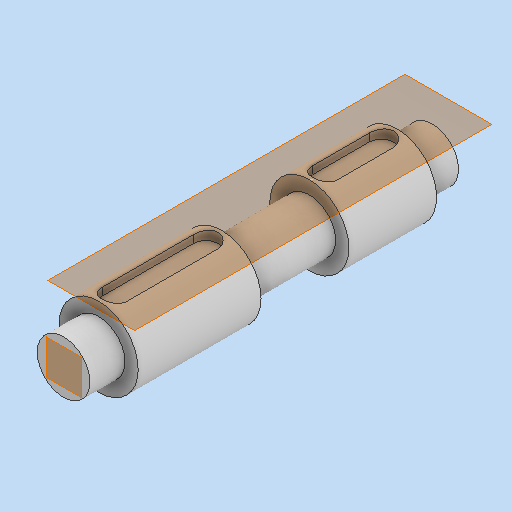
# Autodesk Inventor part: shift2
Saved by Autodesk Inventor 2022 (Build 260153000, 153)
## iProperties
Created: 2023-12-21
Part Number: shift2
Material: 一般
Document SubType Name: Modeling
Designer: ktamu
Density: 1 g/cm^3
Appearance: 既定
Author: ktamu
Autodesk Inventor part; units mm, degrees
ref_plane "YZ Plane" through (0, 0, 0) normal (1, 0, 0) x (0, 1, 0)
sketch "スケッチ1" plane through (0, 0, 0) normal (0, 0, 1) x (1, 0, 0)
  point P0 (0, 0)
ref_plane "作業平面1" through (0, 0, 45) normal (0, 0, 1) x (1, 0, 0)
ref_plane "作業平面2" through (0, 0, 155) normal (0, 0, 1) x (1, 0, 0)
ref_plane "作業平面3" through (0, 0, 210) normal (0, 0, 1) x (1, 0, 0)
sketch "スケッチ2" plane through (0, 0, 45) normal (0, 0, 1) x (1, 0, 0)
  circle A0 centre (0, 0) radius 22.5
  dimension "d3" = 45
  constraints: 1 centre point, 1 coincident
  measures "d3" diameter of A0
extrude "押し出し1" add sketch "スケッチ2" along normal blind 25
sketch "スケッチ3" plane through (0, 0, 155) normal (0, 0, 1) x (1, 0, 0)
  circle A0 centre (0, 0) radius 22.5
  dimension "d6" = 45
  constraints: 1 centre point, 1 coincident
  measures "d6" diameter of A0
extrude "押し出し2" add sketch "スケッチ3" along normal blind 35
ref_plane "作業平面5" through (0, 22.5, 0) normal (0, 1, 0) x (-1, 0, 0)
sketch "スケッチ5" plane through (0, 22.5, 0) normal (0, 1, 0) x (-1, 0, 0)
  line L0 (22.5, 45) -> (-22.5, 45) projected
  line L1 (0, 45) -> (0, 65)
  line L2 (0, 65) -> (0, 61)
  arc A0 (7, 61) -> (-7, 61) centre (0, 61) ccw
  line L3 (7, 61) -> (7, 45)
  line L4 (7, 45) -> (-7, 45)
  line L5 (-7, 61) -> (-7, 45)
  line L6 (7, 45) -> (-7, 45)
  point P0 (0, 0)
  point P1 (-4, 61)
  dimension "d11" = 20
  dimension "d12" = 4
  dimension "d13" = 7
  constraints: 12 end point, 3 point on circle, 3 point on line, 1 centre point, 1 coincident, 1 collinear, 1 midpoint, 1 perpendicular, 1 vertical
  measures "d11" distance of L1.start L1.end
  measures "d12" distance of L1.end L2.end
  measures "d13" radius of A0
extrude "押し出し3" cut sketch "スケッチ5" against normal blind 5.5
mirror "ミラー1" about plane through (0, 0, 45) normal (0, 0, 1) of "押し出し1", "押し出し3"
sketch "スケッチ6" plane through (0, 22.5, 0) normal (0, 1, 0) x (-1, 0, 0)
  line L0 (22.5, 155) -> (-22.5, 155) projected
  line L1 (0, 155) -> (0, 185)
  line L2 (0, 185) -> (0, 181)
  arc A0 (7, 181) -> (-7, 181) centre (0, 181) ccw
  line L3 (7, 181) -> (7, 155)
  line L4 (-7, 155) -> (-7, 181)
  line L5 (7, 155) -> (-7, 155)
  point P0 (0, 0)
  dimension "d16" = 30
  dimension "d17" = 4
  dimension "d18" = 7
  constraints: 10 end point, 3 point on line, 2 point on circle, 1 centre point, 1 coincident, 1 collinear, 1 midpoint, 1 parallel, 1 perpendicular, 1 vertical
  measures "d16" distance of L1.start L1.end
  measures "d17" distance of L1.end L2.end
  measures "d18" radius of A0
extrude "押し出し4" cut sketch "スケッチ6" against normal blind 5.5
mirror "ミラー2" about plane through (0, 0, 155) normal (0, 0, -1) of "押し出し4", "押し出し2"
sketch "スケッチ7" plane through (0, 0, 0) normal (0, 0, 1) x (1, 0, 0)
  circle A0 centre (0, 0) radius 15
  dimension "d21" = 30
  constraints: 1 centre point, 1 coincident
  measures "d21" diameter of A0
extrude "押し出し5" add sketch "スケッチ7" along normal blind 210
